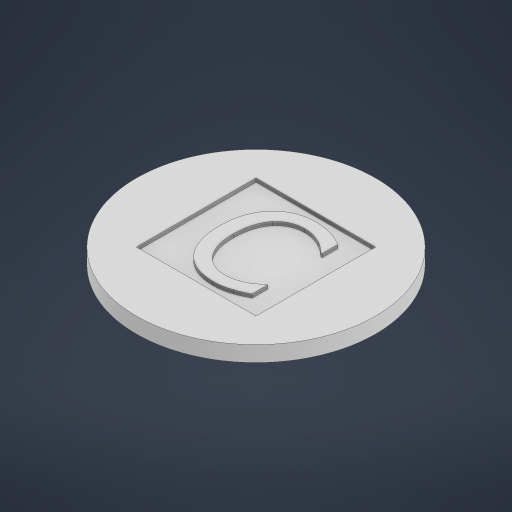
# Autodesk Inventor part: TopMarkerPreset
Saved by Autodesk Inventor 2023.2 (Build 272271030, 271C)
## iProperties
Created: 2023-05-05
Part Number: TopMarkerPreset
Material: Generic
Document SubType Name: Modeling
Designer: Elias Braun
Density: 1 g/cm^3
Appearance: Default
Author: Elias Braun
Autodesk Inventor part; units mm, degrees
ref_plane "YZ Plane" through (0, 0, 0) normal (1, 0, 0) x (0, 1, 0)
ref_plane "XZ Plane" through (0, 0, 0) normal (0, 1, 0) x (-1, 0, 0)
ref_plane "XY Plane" through (0, 0, 0) normal (0, 0, 1) x (1, 0, 0)
sketch "Sketch1" plane through (0, 0, 0) normal (0, 1, 0) x (-1, 0, 0)
  circle A0 centre (0, 0) radius 20
  dimension "d0" = 40
  constraints: 1 centre point, 1 coincident
  measures "d0" diameter of A0
extrude "Extrusion1" add sketch "Sketch1" along normal blind 2.6
sketch "Sketch2" plane through (0, 2.6, 0) normal (0, 1, 0) x (1, 0, 0)
  line L0 (-10, -10) -> (-10, 10)
  line L1 (-10, 10) -> (10, 10)
  line L2 (10, 10) -> (10, -10)
  line L3 (10, -10) -> (-10, -10)
  line L4 (-10, -10) -> (10, 10) construction
  line L5 (-10, 10) -> (10, -10) construction
  point P0 (0, 0)
  dimension "d3" = 20
  dimension "d4" = 20
  constraints: 12 end point, 2 midpoint, 2 parallel, 1 perpendicular, 1 vertical
  measures "d3" distance of L0.start L0.end
  measures "d4" distance of L0.end L1.end
extrude "Extrusion2" cut sketch "Sketch2" against normal blind 0.6
sketch "Sketch3" plane through (0, 2, 0) normal (0, 1, 0) x (1, 0, 0)
  line L0 (-6.8539, 8.6323) -> (6.8539, 8.6323) construction
  line L1 (6.8539, 8.6323) -> (6.8539, -8.5596) construction
  line L2 (6.8539, -8.5596) -> (-6.8539, -8.5596) construction
  line L3 (-6.8539, -8.5596) -> (-6.8539, 8.6323) construction
  spline S0 degree 2 poles (1.3116, -8.5596) (-0.3027, -8.5596) (-3.0335, -7.47) (-4.0289, -6.3803) knots 0 0 0 1 2 2 2
  spline S1 degree 2 poles (-4.0289, -6.3803) (-5.0244, -5.3042) (-6.114, -2.0756) (-6.114, 0.0229) knots 0 0 0 1 2 2 2
  spline S2 degree 2 poles (-6.114, 0.0229) (-6.114, 2.108) (-5.0513, 5.202) (-4.0424, 6.3454) knots 0 0 0 1 2 2 2
  spline S3 degree 2 poles (-4.0424, 6.3454) (-3.0469, 7.462) (-0.3296, 8.6323) (1.3519, 8.6323) knots 0 0 0 1 2 2 2
  spline S4 degree 2 poles (1.3519, 8.6323) (2.186, 8.6323) (3.6523, 8.3902) (4.2711, 8.2018) knots 0 0 0 1 2 2 2
  spline S5 degree 2 poles (4.2711, 8.2018) (4.8092, 8.027) (5.9257, 7.5292) (6.4772, 7.2333) knots 0 0 0 1 2 2 2
  line L4 (6.4772, 7.2333) -> (6.4772, 4.5697)
  line L5 (6.4772, 4.5697) -> (6.3024, 4.5697)
  spline S6 degree 2 poles (6.3024, 4.5697) (6.0064, 4.8388) (5.0917, 5.5921) (4.4325, 5.9553) knots 0 0 0 1 2 2 2
  spline S7 degree 2 poles (4.4325, 5.9553) (3.8002, 6.3051) (2.3071, 6.749) (1.3385, 6.749) knots 0 0 0 1 2 2 2
  spline S8 degree 2 poles (1.3385, 6.749) (0.2758, 6.749) (-1.621, 5.8746) (-2.334, 5.0406) knots 0 0 0 1 2 2 2
  spline S9 degree 2 poles (-2.334, 5.0406) (-3.0335, 4.1931) (-3.8137, 1.6237) (-3.8137, 0.0229) knots 0 0 0 1 2 2 2
  spline S10 degree 2 poles (-3.8137, 0.0229) (-3.8137, -1.6855) (-2.9931, -4.1473) (-2.2801, -4.9948) knots 0 0 0 1 2 2 2
  spline S11 degree 2 poles (-2.2801, -4.9948) (-1.5806, -5.8153) (0.2892, -6.6494) (1.3385, -6.6494) knots 0 0 0 1 2 2 2
  spline S12 degree 2 poles (1.3385, -6.6494) (2.2936, -6.6494) (3.9213, -6.1786) (4.5536, -5.8288) knots 0 0 0 1 2 2 2
  spline S13 degree 2 poles (4.5536, -5.8288) (5.1589, -5.479) (6.0602, -4.7526) (6.3158, -4.497) knots 0 0 0 1 2 2 2
  line L6 (6.3158, -4.497) -> (6.4772, -4.497)
  line L7 (6.4772, -4.497) -> (6.4772, -7.1337)
  spline S14 degree 2 poles (6.4772, -7.1337) (5.9257, -7.3893) (4.9571, -7.8601) (4.2711, -8.0753) knots 0 0 0 1 2 2 2
  spline S15 degree 2 poles (4.2711, -8.0753) (3.5447, -8.3175) (2.3071, -8.5596) (1.3116, -8.5596) knots 0 0 0 1 2 2 2
  point P0 (0, 0)
  constraints: 2 other
extrude "Extrusion3" add sketch "Sketch3" along normal blind 0.6
body "Solid1"
